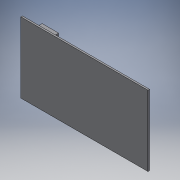
# Autodesk Inventor part: stm32f429
Saved by Autodesk Inventor 2017 (Build 210142000, 142)
## iProperties
Created: 2017-04-25
Part Number: stm32f429
Material: Ogólny
Document SubType Name: Modeling
Designer: Speed King
Density: 1 g/cm^3
Appearance: Domyślna
Mass: 35.596 g
Surface Area: 225.28 cm^2
Volume: 35.596 cm^3
Author: Speed King
Autodesk Inventor part; units mm, degrees
note: some values were not read from the file. Chosen so that the rebuilt part matches the saved one: second side of "Wyciągnięcie proste4".
ref_plane "YZ Plane" through (0, 0, 0) normal (1, 0, 0) x (0, 1, 0)
ref_plane "XZ Plane" through (0, 0, 0) normal (0, 1, 0) x (-1, 0, 0)
ref_plane "XY Plane" through (0, 0, 0) normal (0, 0, 1) x (1, 0, 0)
sketch "Szkic1" plane through (0, 0, 0) normal (0, 1, 0) x (-1, 0, 0)
  line L0 (-59.65, -33) -> (59.65, -33)
  line L1 (59.65, -33) -> (59.65, 33)
  line L2 (59.65, 33) -> (-59.65, 33)
  line L3 (-59.65, 33) -> (-59.65, -33)
  line L4 (-59.65, -33) -> (59.65, 33) construction
  line L5 (59.65, -33) -> (-59.65, 33) construction
  point P0 (0, 0)
  dimension "d0" = 119.3
  dimension "d1" = 66
  constraints: 12 end point, 2 midpoint, 2 parallel, 1 horizontal, 1 perpendicular
  measures "d0" distance of L2.end L1.end
  measures "d1" distance of L1.end L0.end
extrude "Wyciągnięcie proste1" add sketch "Szkic1" along normal blind 1.5
sketch "Szkic3" plane through (0, 1.5, 0) normal (0, 1, 0) x (1, 0, 0)
  line L0 (54.15, -28) -> (-24.59, -28)
  line L1 (-24.59, -28) -> (-24.59, -23)
  line L2 (-24.59, -23) -> (54.15, -23)
  line L3 (54.15, -23) -> (54.15, -28)
  line L4 (-59.65, -33) -> (59.65, -33) projected
  line L5 (59.65, -33) -> (59.65, 33) projected
  line L6 (83.51, 0) -> (-83.51, 0) projected
  point P0 (0, 0)
  dimension "d9" = 78.74
  dimension "d10" = 5
  dimension "d11" = 5
  dimension "d12" = 5.5
  constraints: 8 end point, 2 parallel, 1 horizontal, 1 perpendicular
  measures "d9" distance of L1.end L2.end
  measures "d10" distance between parallel lines of L2 L0
  measures "d11" distance between parallel lines of L0 L4
  measures "d12" distance between parallel lines of L5 L3
extrude "Wyciągnięcie proste6" add sketch "Szkic3" along normal blind 5
sketch "Szkic4" plane through (0, 1.5, 0) normal (0, 1, 0) x (1, 0, 0)
  line L0 (-34.15, -25.5) -> (-49.65, -25.5)
  line L1 (-49.65, -25.5) -> (-49.65, -28)
  line L2 (-49.65, -28) -> (-34.15, -28)
  line L3 (-34.15, -28) -> (-34.15, -25.5)
  line L4 (-59.65, -33) -> (59.65, -33) projected
  line L5 (-59.65, 33) -> (-59.65, -33) projected
  point P0 (0, 0)
  dimension "d17" = 15.5
  dimension "d18" = 2.5
  dimension "d61" = 10
  dimension "d62" = 5
  constraints: 8 end point, 2 parallel, 1 horizontal, 1 perpendicular
  measures "d17" distance of L2.end L1.end
  measures "d18" distance of L1.end L0.end
  measures "d61" distance between parallel lines of L1 L5
  measures "d62" distance between parallel lines of L4 L2
extrude "Wyciągnięcie proste4" add sketch "Szkic4" along normal blind 8.5
sketch "Szkic5" plane through (0, 1.5, 0) normal (0, 1, 0) x (1, 0, 0)
  line L0 (53.65, 21) -> (-6.35, 21)
  line L1 (-6.35, 21) -> (-6.35, -21.5)
  line L2 (-6.35, -21.5) -> (53.65, -21.5)
  line L3 (53.65, -21.5) -> (53.65, 21)
  line L4 (53.65, 21) -> (-6.35, -21.5) construction
  line L5 (-6.35, 21) -> (53.65, -21.5) construction
  line L6 (59.65, -33) -> (59.65, 33) projected
  line L7 (-59.65, -33) -> (59.65, -33) projected
  point P0 (0, 0)
  point P1 (23.65, -0.25)
  dimension "d25" = 60
  dimension "d26" = 42.5
  dimension "d28" = 6
  dimension "d36" = 11.5
  constraints: 12 end point, 2 midpoint, 2 parallel, 1 horizontal, 1 perpendicular
  measures "d25" distance of L2.end L1.end
  measures "d26" distance of L1.end L0.end
  measures "d28" distance from line of L2.end L6
  measures "d36" distance from line of L1.end L7
extrude "Wyciągnięcie proste5" add sketch "Szkic5" along normal blind 5
pattern_linear "Szyk prostokątny1" count 2 spacing 50.5 along (0, 0, -1) of "Wyciągnięcie proste6"
sketch "Szkic6" plane through (0, 1.5, 0) normal (0, 1, 0) x (1, 0, 0)
  line L0 (-51.15, -4) -> (-61.15, -4)
  line L1 (-61.15, -4) -> (-61.15, 5)
  line L2 (-61.15, 5) -> (-51.15, 5)
  line L3 (-51.15, 5) -> (-51.15, -4)
  line L4 (-51.15, -4) -> (-61.15, 5) construction
  line L5 (-61.15, -4) -> (-51.15, 5) construction
  line L6 (-59.65, -33) -> (59.65, -33) projected
  line L7 (-59.65, 33) -> (-59.65, -33) projected
  point P0 (0, 0)
  point P1 (-56.15, 0.5)
  dimension "d37" = 10
  dimension "d38" = 9
  dimension "d39" = 29
  dimension "d40" = 1.5
  constraints: 12 end point, 2 midpoint, 2 parallel, 1 horizontal, 1 perpendicular
  measures "d37" distance of L1.end L2.end
  measures "d38" distance of L0.end L1.end
  measures "d39" distance between parallel lines of L6 L0
  measures "d40" distance from line of L7 L0.end
extrude "Wyciągnięcie proste7" add sketch "Szkic6" along normal blind 5
sketch "Szkic7" plane through (0, 1.5, 0) normal (0, 1, 0) x (1, 0, 0)
  circle A0 centre (-23.65, -13) radius 2.75
  line L0 (-59.65, 33) -> (-59.65, 5) projected
  circle A1 centre (-23.65, 12.5) radius 2.75
  line L1 (-59.65, -33) -> (59.65, -33) projected
  point P0 (0, 0)
  dimension "d43" = 5.5
  dimension "d46" = 25.5
  dimension "d51" = 20
  dimension "d52" = 36
  constraints: 2 centre point, 1 vertical, 2 other
  measures "d43" diameter of A0
  measures "d46" distance of A0.centre A1.centre
  measures "d51" distance from line of L1 A0.centre
  measures "d52" distance from line of A0.centre L0
extrude "Wyciągnięcie proste8" add sketch "Szkic7" along normal blind 10.5
sketch "Szkic8" plane through (0, 1.5, 0) normal (0, 1, 0) x (1, 0, 0)
  line L0 (-32.65, -17.5) -> (-48.15, -17.5)
  line L1 (-48.15, -17.5) -> (-48.15, 27)
  line L2 (-48.15, 27) -> (-32.65, 27)
  line L3 (-32.65, 27) -> (-32.65, -17.5)
  line L4 (-32.65, -17.5) -> (-48.15, 27) construction
  line L5 (-48.15, -17.5) -> (-32.65, 27) construction
  line L6 (-59.65, -33) -> (59.65, -33) projected
  line L7 (-59.65, -4) -> (-59.65, -33) projected
  point P0 (0, 0)
  point P1 (-40.4, 4.75)
  dimension "d55" = 15.5
  dimension "d56" = 27
  dimension "d57" = 44.5
  dimension "d58" = 15.5
  constraints: 12 end point, 2 midpoint, 2 parallel, 1 horizontal, 1 perpendicular
  measures "d55" distance between parallel lines of L6 L0
  measures "d56" distance between parallel lines of L7 L3
  measures "d57" distance of L2.end L0.start
  measures "d58" distance of L0.start L0.end
extrude "Wyciągnięcie proste9" add sketch "Szkic8" along normal blind 8
